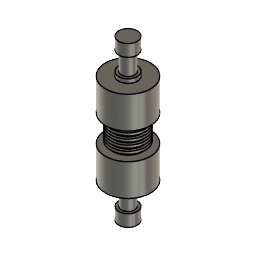
Roller 2 (Autodesk Fusion 360 design; units mm, degrees)
Autodesk Fusion 360 part; units mm, degrees
sketch "Sketch1" plane through (0, 0, 0) normal (0, 0, 1) x (1, 0, 0)
  circle A0 centre (0, 0) radius 3.5
  circle A1 centre (0, 0) radius 8.5
  circle A2 centre (0, 0) radius 2.5
  circle A3 centre (0, 0) radius 6.5
  circle A4 centre (0, 0) radius 5.5
  dimension "d1" = 7
  dimension "d2" = 5
  dimension "d10" = -1
  dimension "d17" = -2
  dimension "d21" = -1
  constraint coincident A0.centre A1.centre
  measures "d1" diameter of A0
extrude "Extrude1" add sketch "Sketch1" along normal blind 60 contours A0 | A1 | A2 | A3 | A4
extrude "Extrude2" cut sketch "Sketch1" along normal blind 13 contours A1 | A3 | A4
extrude "Extrude3" cut sketch "Sketch1" against normal blind 13 from surface at 60 contours A1 | A3 | A4
extrude "Extrude4" cut sketch "Sketch1" along normal blind 7 from surface at 4.5 contours A0
extrude "Extrude5" cut sketch "Sketch1" against normal blind 7 from surface at 55.5 contours A0
extrude "Extrude6" cut sketch "Sketch1" along normal blind 10 from surface at 25 contours A1
extrude "Extrude7" cut sketch "Sketch1" along normal blind 1 from surface at 25 contours A3
extrude "Extrude8" cut sketch "Sketch1" along normal blind 1 from surface at 27 contours A3
extrude "Extrude9" cut sketch "Sketch1" along normal blind 1 from surface at 29 contours A3
extrude "Extrude10" cut sketch "Sketch1" along normal blind 1 from surface at 31 contours A3
extrude "Extrude11" cut sketch "Sketch1" along normal blind 1 from surface at 33 contours A3
